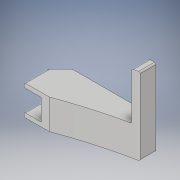
# Autodesk Inventor part: CH_01_0024_piston_adapter
Saved by Autodesk Inventor 2019 (Build 230136000, 136)
## iProperties
Created: 2022-03-04
Part Number: CH_01_0024_piston_adapter
Material: Ogólny
Document SubType Name: Modeling
Designer: zsamot8
Density: 1 g/cm^3
Appearance: Domyślna
Author: zsamot8
Autodesk Inventor part; units mm, degrees
ref_plane "YZ Plane" through (0, 0, 0) normal (1, 0, 0) x (0, 1, 0)
ref_plane "XZ Plane" through (0, 0, 0) normal (0, 1, 0) x (-1, 0, 0)
ref_plane "XY Plane" through (0, 0, 0) normal (0, 0, 1) x (1, 0, 0)
sketch "Szkic1" plane through (0, 0, 0) normal (0, 0, 1) x (1, 0, 0)
  line L0 (0, 0) -> (0, 33.1)
  line L1 (0, 33.1) -> (5, 33.1)
  line L2 (5, 33.1) -> (5, -21)
  line L3 (-62.5, -3) -> (-62.5, 0)
  line L4 (-62.5, 0) -> (0, 0)
  line L5 (-62.5, -3) -> (-50.5, -3)
  line L6 (-50.5, -3) -> (-50.5, -18)
  line L7 (-50.5, -18) -> (-62.5, -18)
  line L8 (-62.5, -18) -> (-62.5, -21)
  line L9 (-62.5, -21) -> (5, -21)
  dimension "d1" = 15
  dimension "d3" = 3
  dimension "d4" = 12
  dimension "d6" = 3
  dimension "d7" = 5
  dimension "d8" = 33.1
  dimension "d9" = 50.5
  constraints: 20 end point, 6 perpendicular, 1 collinear, 1 horizontal, 1 vertical
  measures "d1" distance between parallel lines of L5 L7
  measures "d3" distance between parallel lines of L7 L9
  measures "d4" distance between parallel lines of L3 L6
  measures "d6" distance between parallel lines of L4 L5
  measures "d7" distance between parallel lines of L2 L0
  measures "d8" distance between parallel lines of L4 L1
  measures "d9" distance between parallel lines of L6 L0
extrude "Wyciągnięcie proste1" add sketch "Szkic1" along normal blind 25
sketch "Szkic2" plane through (-50.5, -18, 0) normal (-1, 0, 0) x (0, 0, 1)
  line L0 (0, 0) -> (0, 15) construction
  line L1 (0, 0) -> (25, 0) construction
  line L2 (25, 15) -> (25, 0) construction
  line L3 (0, 15) -> (25, 15) construction
  line L4 (0, 15) -> (12, 15)
  line L5 (12, 15) -> (12, 0)
  line L6 (12, 0) -> (0, 0)
  line L7 (0, 0) -> (0, 15)
  point P0 (0, 18)
  dimension "d14" = 13
  constraints: 8 end point, 2 parallel, 1 horizontal, 1 perpendicular, 1 point on line
  measures "d14" distance between parallel lines of L2 L5
extrude "Wyciągnięcie proste2" add sketch "Szkic2" along normal up to surface (12 mm away)
chamfer "Faza1" distance 9 angle 45 1 edges at (-62.5, -10.5, 0)
sketch "Szkic4" plane through (-62.5, -21, 25) normal (0, -1, 0) x (1, 0, 0)
  line L0 (0, 0) -> (67.5, 0) construction
  line L1 (62.5, 0) -> (0, 0) construction
  arc A0 (17.5, 0) -> (67.5, -14) centre (131.2021, 309.7932) ccw
  line L2 (67.5, 0) -> (67.5, -25) construction
  line L3 (62.5, -25) -> (67.5, -25) construction
  line L4 (17.5, 0) -> (67.5, 0)
  line L5 (67.5, 0) -> (67.5, -14)
  dimension "d21" = 11
  dimension "d23" = 50
  dimension "d24" = 330
  constraints: 8 end point, 2 point on circle, 2 point on line, 1 centre point, 1 collinear, 1 horizontal, 1 perpendicular, 1 vertical
  measures "d21" distance of L5.end L2.end
  measures "d23" distance from line of L2 L4.start
  measures "d24" radius of A0
extrude "Wyciągnięcie proste3" cut sketch "Szkic4" against normal up to surface (54.1 mm away)
fillet "Zaokrąglenie1" radius 1 8 edges at (5, -21, 5.5) (0, 0, 6.012) (5, 33.1, 5.5) (0, 33.1, 6.012) (-62.5, 0, 17) (-62.5, -21, 17) (-62.5, -18, 18.5) (-62.5, -3, 18.5)
equation "\"d3\" = d2"
equation "\"d2\" = 3"
